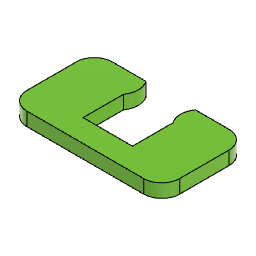
Switch_Slider_Clamp_M2 (Autodesk Fusion 360 design; units mm, degrees)
Autodesk Fusion 360 part; units mm, degrees
sketch "Skizze1" plane through (0, 0, 0) normal (0, 0, 1) x (1, 0, 0)
  line L0 (6.5, -4.75) -> (-6.5, -4.75)
  line L1 (-8.5, -2.75) -> (-8.5, 2.75)
  line L2 (-6.5, 4.75) -> (6.5, 4.75)
  line L3 (8.5, 2.75) -> (8.5, -2.75)
  line L4 (8.5, -4.75) -> (-8.5, 4.75) construction
  line L5 (-8.5, -4.75) -> (8.5, 4.75) construction
  arc A0 (-6.5, 4.75) -> (-8.5, 2.75) centre (-6.5, 2.75) ccw
  arc A1 (8.5, 2.75) -> (6.5, 4.75) centre (6.5, 2.75) ccw
  arc A2 (6.5, -4.75) -> (8.5, -2.75) centre (6.5, -2.75) ccw
  arc A3 (-8.5, -2.75) -> (-6.5, -4.75) centre (-6.5, -2.75) ccw
  line L6 (2.75, -2.25) -> (-2.75, -2.25)
  line L7 (-2.75, -2.25) -> (-2.75, 2.25)
  line L8 (-2.75, 2.25) -> (2.75, 2.25)
  line L9 (2.75, 2.25) -> (2.75, -2.25)
  line L10 (2.75, -2.25) -> (-2.75, 2.25) construction
  line L11 (-2.75, -2.25) -> (2.75, 2.25) construction
  line L12 (-2.75, 2.25) -> (-2.75, 4.75)
  line L13 (2.75, 2.25) -> (2.75, 4.75)
  arc A4 (-2.75, 2.25) -> (-2.75, 4.75) centre (-4.5, 3.5) ccw
  arc A5 (2.75, 4.75) -> (2.75, 2.25) centre (4.5, 3.5) ccw
  dimension "d487" = 17
  dimension "d488" = 9.5
  dimension "d489" = 2
  dimension "d491" = 5.5
  dimension "d492" = 4.5
  dimension "d501" = 9
  constraint horizontal L0
  constraint perpendicular L0 L1
  constraint parallel L0 L2
  constraint parallel L1 L3
  constraint coincident L4 origin
  constraint coincident L5 origin
  constraint coincident L4.end L1
  constraint coincident L4.end L2
  constraint tangent L1 A0
  constraint tangent L2 A0
  constraint coincident L5.end L2
  constraint coincident L5.end L3
  constraint tangent L2 A1
  constraint tangent L3 A1
  constraint equal A0 A1
  constraint coincident L4.start L3
  constraint coincident L4.start L0
  constraint tangent L3 A2
  constraint tangent L0 A2
  constraint equal A0 A2
  constraint coincident L5.start L0
  constraint coincident L5.start L1
  constraint tangent L0 A3
  constraint tangent L1 A3
  constraint equal A0 A3
  constraint horizontal L6
  constraint perpendicular L6 L7
  constraint parallel L6 L8
  constraint parallel L7 L9
  constraint coincident L10 origin
  constraint coincident L11 origin
  constraint coincident L2 L12.end
  constraint perpendicular L2 L12
  constraint perpendicular L8 L13
  constraint coincident L2 L13.end
  constraint equal A4 A5
  measures "d487" distance of L4.end L5.end
  measures "d488" distance of L5.start L4.end
  measures "d489" radius of A0
  measures "d491" distance of L6.start L6.end
  measures "d492" distance of L6.end L7.end
  measures "d501" distance of A4.centre A5.centre
extrude "Extrusion1" add sketch "Skizze1" along normal blind 1.5 contours L0 L1 L2 L3 A0 A1 A2 A3 L6 L7 L9 L12 L13 | L13 A5 | L12 A4
named bodies: "Switch_Slider_Clamp"
